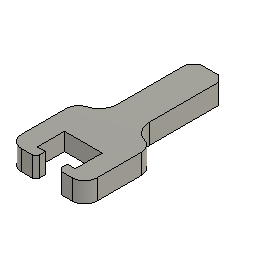
bit_connector_hold_tool (Autodesk Fusion 360 design; units mm, degrees)
Autodesk Fusion 360 part; units mm, degrees
note: some values were not read from the file. Set by a fixed rule: which sketch regions a step uses.
sketch "スケッチ1" plane through (0, 0, 0) normal (0, 0, 1) x (1, 0, 0)
  line L0 (-6, -10.8) -> (-1.75, -10.8)
  line L1 (-1.75, -10.8) -> (-1.75, -9.3)
  line L2 (-1.75, -9.3) -> (-3, -9.3)
  line L3 (-3, -9.3) -> (-3, -5)
  line L4 (-3, -5) -> (3, -5)
  line L5 (3, -5) -> (3, -9.3)
  line L6 (3, -9.3) -> (1.75, -9.3)
  line L7 (1.75, -9.3) -> (1.75, -10.8)
  line L8 (1.75, -10.8) -> (6, -10.8)
  line L9 (6, -10.8) -> (6, 0)
  line L10 (6, 0) -> (5.5, 0)
  line L11 (2.5, 3) -> (2.5, 15)
  line L12 (2.5, 15) -> (-2.5, 15)
  line L13 (-2.5, 15) -> (-2.5, 3)
  line L14 (-5.5, 0) -> (-6, 0)
  line L15 (-6, 0) -> (-6, -10.8)
  line L16 (0, 0) -> (0, -5) construction
  line L17 (-2.5, 0) -> (1.5, 0) construction
  arc A0 (-5.5, 0) -> (-2.5, 3) centre (-5.5, 3) ccw
  arc A1 (2.5, 3) -> (5.5, 0) centre (5.5, 3) ccw
  dimension "d4" = 6
  dimension "d5" = 1.5
  dimension "d6" = 4.3
  dimension "d7" = 3
  dimension "d8" = 5
  dimension "d9" = 5
  dimension "d10" = 15
  dimension "d11" = 3.5
  dimension "d12" = 3
  dimension "d13" = 3
  constraint horizontal L0
  constraint perpendicular L0 L1
  constraint perpendicular L1 L2
  constraint perpendicular L2 L3
  constraint perpendicular L1 L4
  constraint perpendicular L4 L5
  constraint perpendicular L1 L6
  constraint perpendicular L4 L7
  constraint perpendicular L7 L8
  constraint perpendicular L4 L9
  constraint perpendicular L7 L10
  constraint perpendicular L10 L11
  constraint perpendicular L7 L12
  constraint perpendicular L10 L13
  constraint perpendicular L13 L14
  constraint perpendicular L10 L15
  constraint coincident L0.start L15.end
  constraint coincident L16.start origin
  constraint coincident L4 L16.end
  constraint perpendicular L4 L16
  constraint symmetric L3 L5 L16
  constraint symmetric L9 L15 L16
  constraint symmetric L1 L7 L16
  constraint symmetric L0 L8 L16
  constraint symmetric L2 L6 L16
  constraint symmetric L10 L14 L16
  constraint coincident L16.start L17
  constraint coincident L17.start L13
  constraint tangent L13 A0
  constraint tangent L14 A0
  constraint coincident L17.end L10
  constraint tangent L11 A1
  constraint tangent L10 A1
  measures "d4" distance of L3 L5
  measures "d5" distance of L0.end L1.end
  measures "d6" distance of L2.end L3.end
  measures "d7" distance of L5 L9
  measures "d8" distance of L4 L10
  measures "d9" distance of L11 L13
  measures "d10" distance of L12 L14
  measures "d11" distance of L1 L7
  measures "d12" radius of A0
  measures "d13" radius of A1
extrude "押し出し1" add sketch "スケッチ1" along normal blind 3.2
fillet "フィレット1" radius 2 4 edges at (-6, 0, 1.6) (-6, -10.8, 1.6) (6, 0, 1.6) (6, -10.8, 1.6)
chamfer "面取り1" distance 1 angle 45 2 edges at (2.5, 15, 1.6) (-2.5, 15, 1.6)
chamfer "面取り2" distance 0.5 angle 45 2 edges at (1.75, -10.8, 1.6) (-1.75, -10.8, 1.6)
chamfer "面取り3" distance 0.4 angle 45 3 edges at (3, -7.15, 0) (0, -5, 0) (-3, -7.15, 0)
equation "d1 = 3.7 mm - 0.5 mm"
